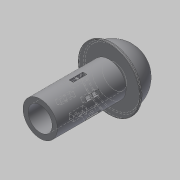
# Autodesk Inventor part: 主體
Saved by Autodesk Inventor 2018 (Build 220112000, 112)
## iProperties
Created: 2021-03-05
Part Number: 主體
Material: 一般
Document SubType Name: Modeling
Designer: 王鼎鈞
Density: 1 g/cm^3
Appearance: 預設
Mass: 319.933 g
Surface Area: 399.291 cm^2
Volume: 319.933 cm^3
Author: 王鼎鈞
Autodesk Inventor part; units mm, degrees
ref_plane "YZ Plane" through (0, 0, 0) normal (1, 0, 0) x (0, 1, 0)
ref_plane "XZ Plane" through (0, 0, 0) normal (0, 1, 0) x (-1, 0, 0)
ref_plane "XY Plane" through (0, 0, 0) normal (0, 0, 1) x (1, 0, 0)
sketch "草圖1" plane through (0, 0, 0) normal (1, 0, 0) x (0, 1, 0)
  line L0 (0, 0) -> (100, 0)
  line L1 (100, 0) -> (100, -25)
  line L2 (100, -25) -> (0, -25)
  line L3 (0, -25) -> (0, 0)
  dimension "d0" = 100
  dimension "d1" = 25
  constraints: 8 end point, 2 parallel, 1 horizontal, 1 perpendicular
  measures "d0" distance of L1.end L2.end
  measures "d1" distance of L0.end L1.end
revolve "迴轉1" add sketch "草圖1" angle 360 about axis through (0, 0, 0) along (0, 1, 0)
sketch "草圖2" plane through (0, 0, 0) normal (1, 0, 0) x (0, 1, 0)
  line L0 (100, 25) -> (100, -25) projected
  line L1 (100, 0) -> (105, 0)
  line L2 (105, 0) -> (105, 45)
  line L3 (105, 45) -> (100, 45)
  line L4 (100, 45) -> (100, 0)
  point P0 (0, 0)
  dimension "d3" = 5
  dimension "d4" = 45
  constraints: 8 end point, 2 parallel, 1 horizontal, 1 midpoint, 1 perpendicular
  measures "d3" distance of L3.end L2.end
  measures "d4" distance of L2.end L1.end
revolve "迴轉2" add sketch "草圖2" angle 360 about axis through (0, 100, 0) along (0, 1, 0)
fillet "圓角1" radius 3 1 edges at (0, 105, -45)
fillet "圓角2" radius 0.5 1 edges at (0, 100, -45)
sketch "草圖3" plane through (0, 0, 0) normal (1, 0, 0) x (0, 1, 0)
  line L0 (105, 42) -> (105, -42) projected
  arc A0 (144.8826, 0) -> (105, 39.8826) centre (105, 0) ccw
  line L1 (144.8826, 0) -> (105, 0)
  point P0 (0, 0)
  constraints: 2 end point, 2 point on circle, 1 centre point, 1 midpoint, 1 perpendicular, 1 point on line
revolve "迴轉3" add sketch "草圖3" angle 360 about axis through (0, 144.8826, 0) along (0, -1, 0)
sketch "草圖4" plane through (0, 0, 0) normal (0, -1, 0) x (1, 0, 0)
  circle A0 centre (0, 0) radius 17.5
  dimension "d9" = 35
  constraints: 1 centre point, 1 coincident
  measures "d9" diameter of A0
extrude "擠出1" cut sketch "草圖4" against normal blind 40
sketch "草圖5" plane through (0, 0, 0) normal (1, 0, 0) x (0, 1, 0)
  line L0 (0, 25) -> (0, -25) projected
  line L1 (100, 25) -> (100, -25) projected
  line L2 (100, 25) -> (0, 25) projected
  arc A0 (53.3486, 19.4954) -> (56.6514, 19.4954) centre (55, 22) ccw
  line L3 (65, 25) -> (56.6514, 19.4954)
  line L4 (45, 25) -> (53.3486, 19.4954)
  circle A1 centre (55, 22) radius 1.5
  line L5 (65, 25) -> (65, 35.073)
  line L6 (65, 35.073) -> (43.5006, 35.585)
  line L7 (43.5006, 35.585) -> (45, 25)
  point P0 (0, 0)
  dimension "d12" = 6
  dimension "d13" = 0
  dimension "d14" = 55
  dimension "d15" = 10
  dimension "d16" = 10
  dimension "d17" = 3
  constraints: 10 end point, 2 centre point, 2 point on circle, 2 point on line, 2 tangent, 1 coincident, 1 vertical
  measures "d12" diameter of A0
  measures "d13" distance edge to line of A0 L2
  measures "d14" distance from line of L0 A0.centre
  measures "d15" horizontal distance of A0.centre L4.start
  measures "d16" horizontal distance of A0.centre L3.start
  measures "d17" diameter of A1
extrude "擠出2" cut sketch "草圖5" along normal mid plane 6
pattern_circular "環形陣列1" count 6 over 360 about axis through (0, -10, 0) along (0, 1, 0) of "擠出2"
sketch "草圖6" plane through (0, 0, 0) normal (1, 0, 0) x (0, 1, 0)
  circle A0 centre (55, -22) radius 1.5 construction
  circle A1 centre (55, 22) radius 1.5 construction
  arc A2 (100.5, 45) -> (100, 44.5) centre (100.5, 44.5) ccw construction
  line L0 (100.5, 45) -> (102, 45) construction
  arc A3 (105, 42) -> (102, 45) centre (102, 42) ccw construction
  line L1 (105, 42) -> (105, 39.8826) construction
  arc A4 (105, -39.8826) -> (144.8826, 0) centre (105, 0) ccw construction
  arc A5 (144.8826, 0) -> (105, 39.8826) centre (105, 0) ccw construction
  line L2 (105, -39.8826) -> (105, -42) construction
  arc A6 (102, -45) -> (105, -42) centre (102, -42) ccw construction
  line L3 (102, -45) -> (100.5, -45) construction
  arc A7 (100, -44.5) -> (100.5, -45) centre (100.5, -44.5) ccw construction
  line L4 (100, -44.5) -> (100, -25) construction
  line L5 (100, -25) -> (65, -25) construction
  line L6 (65, -25) -> (56.6514, -19.4954) construction
  arc A8 (56.6514, -19.4954) -> (53.3486, -19.4954) centre (55, -22) ccw construction
  line L7 (53.3486, -19.4954) -> (45, -25) construction
  line L8 (45, -25) -> (0, -25) construction
  line L9 (0, -25) -> (0, -17.5) construction
  line L10 (0, -17.5) -> (40, -17.5) construction
  line L11 (40, -17.5) -> (40, 17.5) construction
  line L12 (40, 17.5) -> (0, 17.5) construction
  line L13 (0, 17.5) -> (0, 25) construction
  line L14 (0, 25) -> (45, 25) construction
  line L15 (45, 25) -> (53.3486, 19.4954) construction
  arc A9 (53.3486, 19.4954) -> (56.6514, 19.4954) centre (55, 22) ccw construction
  line L16 (56.6514, 19.4954) -> (65, 25) construction
  line L17 (65, 25) -> (100, 25) construction
  line L18 (100, 25) -> (100, 44.5) construction
  arc A10 (140.4436, -10.2017) -> (140.2979, 10.695) centre (105, 0) ccw
  arc A11 (140.2979, -10.695) -> (140.4436, -10.2017) centre (105, 0) ccw
  line L19 (140.2979, -10.695) -> (140.2979, -40.9413)
  line L20 (140.2979, -40.9413) -> (153.5603, -40.9413)
  line L21 (153.5603, -40.9413) -> (152.7715, 46.0582)
  line L22 (140.2979, 10.695) -> (140.2979, 45.4267)
  line L23 (140.2979, 45.4267) -> (152.7715, 46.0582)
  point P0 (0, 0)
  dimension "d23" = 3
  constraints: 10 end point, 4 point on circle, 2 centre point, 2 vertical, 1 collinear, 1 perpendicular
  measures "d23" radial gap between concentric circles of A4 A10
extrude "擠出3" cut sketch "草圖6" along normal mid plane 3
fillet "圓角3" radius 1.5 4 edges at (-1.5, 140.2979, 14.5999) (1.5, 140.2979, 14.5999) (1.5, 140.2979, -14.5999) (-1.5, 140.2979, -14.5999)
sketch "草圖7" plane through (0, 0, 0) normal (1, 0, 0) x (0, 1, 0)
  line L0 (-28.9709, 0) -> (173.8252, 0) projected
  line L1 (0, -63) -> (0, 63) projected
  line L2 (40, -17.5) -> (40, 17.5) projected
  line L3 (107.8583, 0) -> (40, 0)
  line L4 (40, 0) -> (40, 17.5)
  line L5 (40, 17.5) -> (107.8583, 17.5)
  line L6 (107.8583, 17.5) -> (107.8583, 0)
  point P0 (0, 0)
  constraints: 8 end point, 2 parallel, 1 horizontal, 1 perpendicular, 1 point on line
revolve "迴轉4" cut sketch "草圖7" angle 360 about axis through (0, -10, 0) along (0, 1, 0)
sketch "草圖8" plane through (0, 0, 0) normal (1, 0, 0) x (0, 1, 0)
  ellipse E0 centre (82.9167, 0) end of major axis (119.8845, -17.0004) minor radius 20.1752 (45.274, 15.0077) -> (45.274, 9.8116) ccw projected
  line L0 (45.274, 9.8116) -> (64.726, 9.8116) projected
  ellipse E1 centre (27.0833, 0) end of major axis (-9.8845, -17.0004) minor radius 20.1752 (64.726, 9.8116) -> (64.726, 15.0077) ccw projected
  line L1 (64.726, 15.0077) -> (45.274, 15.0077) projected
  ellipse E2 centre (82.9167, 0) end of major axis (45.9489, -17.0004) minor radius 20.1752 (45.274, -9.8116) -> (45.274, -15.0077) ccw projected
  line L2 (45.274, -15.0077) -> (64.726, -15.0077) projected
  ellipse E3 centre (27.0833, 0) end of major axis (64.0511, -17.0004) minor radius 20.1752 (64.726, -15.0077) -> (64.726, -9.8116) ccw projected
  line L3 (64.726, -9.8116) -> (45.274, -9.8116) projected
  line L4 (45.274, -24.8193) -> (45.274, -24.8193) projected
  line L5 (45.274, -24.8193) -> (64.726, -24.8193) projected
  line L6 (64.726, -24.8193) -> (64.726, -24.8193) projected
  line L7 (64.726, -24.8193) -> (45.274, -24.8193) projected
  ellipse E4 centre (82.9167, 0) end of major axis (45.9489, -17.0004) minor radius 20.1752 (45.274, -9.8116) -> (45.274, -15.0077) ccw projected
  line L8 (45.274, -9.8116) -> (64.726, -9.8116) projected
  ellipse E5 centre (27.0833, 0) end of major axis (64.0511, -17.0004) minor radius 20.1752 (64.726, -15.0077) -> (64.726, -9.8116) ccw projected
  line L9 (64.726, -15.0077) -> (45.274, -15.0077) projected
  ellipse E6 centre (82.9167, 0) end of major axis (119.8845, -17.0004) minor radius 20.1752 (45.274, 15.0077) -> (45.274, 9.8116) ccw projected
  line L10 (45.274, 15.0077) -> (64.726, 15.0077) projected
  ellipse E7 centre (27.0833, 0) end of major axis (-9.8845, -17.0004) minor radius 20.1752 (64.726, 9.8116) -> (64.726, 15.0077) ccw projected
  line L11 (64.726, 9.8116) -> (45.274, 9.8116) projected
  line L12 (45.274, 24.8193) -> (45.274, 24.8193) projected
  line L13 (45.274, 24.8193) -> (64.726, 24.8193) projected
  line L14 (64.726, 24.8193) -> (64.726, 24.8193) projected
  line L15 (64.726, 24.8193) -> (45.274, 24.8193) projected
  line L16 (0, 25) -> (0, -25) projected
  line L17 (100, 25) -> (100, -25) projected
  line L18 (100, -25) -> (0, -25) projected
  ellipse E8 centre (27.0833, 0) end of major axis (64.0511, -17.0004) minor radius 20.1752 (64.726, -15.0077) -> (64.726, -9.8116) ccw projected
  line L19 (45.0013, -25) -> (64.9953, -25)
  line L20 (64.9953, -25) -> (64.9953, -12.1579)
  line L21 (64.9953, -12.1579) -> (45.0013, -12.1579)
  line L22 (45.0013, -12.1579) -> (45.0013, -25)
  circle A0 centre (55, -22) radius 1.5 projected
  circle A1 centre (55, -22) radius 1.5 projected
  point P0 (0, 0)
  constraints: 8 end point, 2 parallel, 1 horizontal, 1 perpendicular, 1 point on line, 10 other
extrude "擠出4" cut sketch "草圖8" along normal mid plane 6 contours L21 L20 E3 L2 E2 | E2 L2 E3 L20 L18 L22
pattern_circular "環形陣列2" count 6 over 360 about axis through (0, -10, 0) along (0, 1, 0) of "擠出4"
sketch "草圖9" plane through (0, 0, 0) normal (1, 0, 0) x (0, 1, 0)
  circle A0 centre (55, -22) radius 1.5 projected
  circle A1 centre (55, -22) radius 18.5
  circle A2 centre (55, 22) radius 1.5 projected
  circle A3 centre (55, 22) radius 18.5
  line L0 (0, -17.5) -> (107.8583, -17.5) projected
  line L1 (0, 17.5) -> (107.8583, 17.5) projected
  line L2 (81.619, -17.5) -> (31.619, -17.5)
  line L3 (31.619, -17.5) -> (31.619, 17.5)
  line L4 (31.619, 17.5) -> (81.619, 17.5)
  line L5 (81.619, 17.5) -> (81.619, -17.5)
  point P0 (0, 0)
  dimension "d33" = 37
  dimension "d34" = 37
  dimension "d35" = 50
  constraints: 8 end point, 2 centre point, 2 coincident, 2 parallel, 2 point on line, 1 horizontal, 1 perpendicular
  measures "d33" diameter of A1
  measures "d34" diameter of A3
  measures "d35" distance between parallel lines of L5 L3
delete faces "刪除面1" heal yes whole lump no faces at (-0.5, 141.8798, 0.4494) (0.5, 141.8798, 0.4494) (0.3916, 140.4274, -10.258) (-0.374, 140.4211, -10.2795) (1.4911, 141.6346, -8.0822) (0, 140.2979, -13.3185) (-1.4911, 141.6346, -8.0822) (-0.0001, 140.2979, 13.3185) (1.4905, 141.6291, 8.1115) (-1.4905, 141.6291, 8.1115) (1.5, 142.5595, -8.5368) (-1.5, 142.5595, -8.5368)
